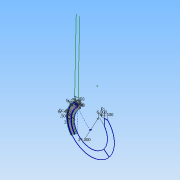
# Autodesk Inventor part: HOT Thermo bulb outline L
Saved by Autodesk Inventor 2013 (Build 170138000, 138)
## iProperties
Created: 2018-07-29
Part Number: HOT Thermo bulb outline L
Material: Generic
Document SubType Name: Modeling
Designer: Jeff Vyduna
Density: 1 g/cm^3
Author: Jeff Vyduna
Autodesk Inventor part; units mm, degrees
ref_plane "YZ Plane" through (0, 0, 0) normal (1, 0, 0) x (0, 1, 0)
ref_plane "XZ Plane" through (0, 0, 0) normal (0, 1, 0) x (-1, 0, 0)
ref_plane "XY Plane" through (0, 0, 0) normal (0, 0, 1) x (1, 0, 0)
ref_plane "Work Plane1" through (22.5184, 2.463, -18.3509) normal (0, 0, 1) x (0.9997722, -0.0213418, 0)
sketch "ThermoBulbBorder" plane through (22.5184, 2.463, -18.3509) normal (0, 0, 1) x (0.9997722, -0.0213418, 0)
  arc A0 (-447.455, -468.958) -> (162.145, -468.958) centre (-142.655, -774.8145) ccw
  arc A1 (-339.505, -542.1063) -> (98.645, -588.5959) centre (-142.655, -774.8145) ccw
  line L0 (-447.455, -468.958) -> (-339.505, -468.958)
  line L1 (162.145, -468.958) -> (98.645, -468.958)
  line L2 (98.645, -468.958) -> (98.645, -588.5959)
  line L3 (-383.955, -961.033) -> (-484.4967, -1038.6241)
  line L4 (98.645, -961.033) -> (199.1867, -1038.6241)
  arc A2 (-447.455, -468.958) -> (162.145, -468.958) centre (-142.655, -774.8145) ccw projected
  line L5 (98.645, -468.958) -> (98.645, -316.558) construction
  line L6 (-339.505, -468.958) -> (-339.505, -542.1063)
  line L7 (-383.955, -468.958) -> (-383.955, 914.2855) projected
  line L8 (-447.455, 914.2855) -> (-447.455, -468.958) projected
  line L9 (-383.955, -468.958) -> (-383.955, -961.033) construction
  dimension "d0" = 609.6
  dimension "d6" = 63.5
  dimension "d12" = 152.4
  dimension "d53" = 107.95
  constraints: 16 end point, 8 point on circle, 3 vertical, 2 centre point, 2 horizontal, 2 line through centre, 1 coincident, 1 collinear, 1 concentric, 1 horizontal alignment, 1 vertical alignment
  measures "d0" diameter of A1
  measures "d6" distance of L1.start L1.end
  measures "d12" distance of L1.end L5.end
  measures "d53" distance of L0.end L0.start
extrude "Extrusion6" add sketch "ThermoBulbBorder" along normal blind 18.034 contours L0 L6 A1 L3 A0
sketch "Sketch3" plane through (22.5184, 2.463, -0.3169) normal (0, 0, 1) x (0.9997722, -0.0213418, 0)
  arc A0 (-447.455, -468.958) -> (-484.4967, -1038.6241) centre (-142.655, -774.8145) ccw projected
  line L0 (-484.4967, -1038.6241) -> (-383.955, -961.033) projected
  arc A1 (-339.505, -542.1063) -> (-383.955, -961.033) centre (-142.655, -774.8145) ccw projected
  line L1 (-339.505, -468.958) -> (-447.455, -468.958) projected
  arc A2 (-429.1801, -468.958) -> (-435.8114, -475.308) centre (-142.655, -774.8145) ccw construction
  arc A3 (-436.6135, -493.4561) -> (-464.7905, -1023.4163) centre (-142.655, -774.8145) ccw
  line L2 (-474.4425, -1030.865) -> (-464.7905, -1023.4163)
  arc A4 (-373.4379, -528.461) -> (-409.8948, -981.0515) centre (-142.655, -774.8145) ccw
  line L3 (-142.655, -774.8145) -> (-429.1801, -468.958) construction
  line L4 (-419.5468, -988.5003) -> (-409.8948, -981.0515)
  line L5 (-396.3065, -475.308) -> (-422.6679, -475.308)
  line L6 (-422.6679, -487.5) -> (-396.2592, -487.5)
  arc A5 (-445.4213, -485.0259) -> (-474.4425, -1030.865) centre (-142.655, -774.8145) ccw
  arc A6 (-381.7732, -519.5633) -> (-396.2592, -487.5) centre (-396.2592, -506.804) ccw
  arc A7 (-373.4379, -528.461) -> (-396.3065, -475.308) centre (-396.3065, -506.804) ccw
  arc A8 (-422.6679, -487.5) -> (-436.6135, -493.4561) centre (-422.6679, -506.804) ccw
  arc A9 (-422.6679, -475.308) -> (-445.4213, -485.0259) centre (-422.6679, -506.804) ccw
  arc A10 (-381.7732, -519.5633) -> (-419.5468, -988.5003) centre (-142.655, -774.8145) ccw
  point P0 (-22.4607, -2.943)
  point P1 (-383.955, -468.958)
  point P2 (-430.7947, -487.5)
  dimension "d56" = 12.7
  dimension "d57" = 12.192
  dimension "d61" = 63.5
  dimension "d62" = 6.35
  dimension "d63" = 12.192
  dimension "d64" = 19.304
  dimension "d65" = 31.496
  dimension "d66" = 19.304
  dimension "d67" = 31.496
  dimension "d68" = 57.15
  dimension "d69" = 12.192
  constraints: 20 point on circle, 10 end point, 10 point on line, 9 centre point, 6 tangent, 4 coincident, 1 collinear, 1 horizontal, 1 parallel
  measures "d56" radial gap between concentric circles of A0 A2
  measures "d57" radial gap between concentric circles of A2 A3
  measures "d61" distance of point (-383.955, -468.958) L1.end
  measures "d62" distance between parallel lines of L1 L5
  measures "d63" distance between parallel lines of L5 L6
  measures "d64" radius of A6
  measures "d65" radius of A7
  measures "d66" radius of A8
  measures "d67" radius of A9
  measures "d68" radial gap between concentric circles of A10 A3
  measures "d69" radial gap between concentric circles of A10 A4
extrude "Extrusion7" cut sketch "Sketch3" against normal blind 12.7 contours A5 A9 L5 A7 A4 L0 A10 A6 L6 A8 A3
equation "\"d6\" = d5"
equation "\"d57\" = bRopeChannel"
equation "\"d63\" = bRopeChannel"
equation "\"d69\" = bRopeChannel"
equation "\"bRopeChannel\" = 12.192"
equation "\"d8\" = bRopeChannel"
equation "\"d9\" = bRopeChannel"
equation "\"d38\" = bRopeChannel"
equation "\"d60\" = bRopeChannel"
equation "\"d5\" = 63.5"
body "Solid2"
body "Solid3"
